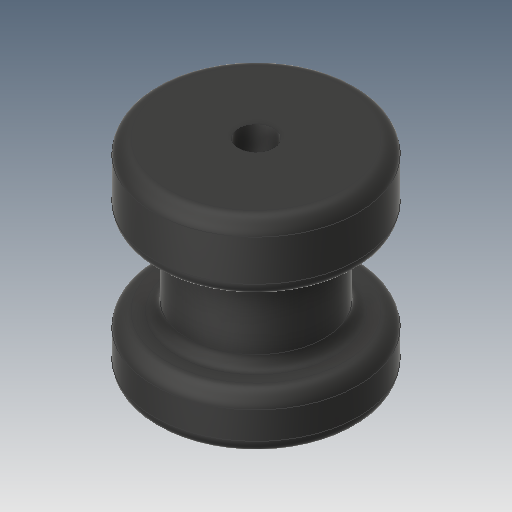
# Autodesk Inventor part: End_Effector_Coupler
Saved by Autodesk Inventor 2020.3 (Build 243373000, 373)
## iProperties
Created: 2021-08-25
Part Number: End_Effector_Coupler
Material: ABS Plastic
Document SubType Name: Modeling
Designer: justi
Density: 1.06 g/cm^3
Appearance: Smooth - Black
Mass: 16.3412 g
Surface Area: 49.2182 cm^2
Volume: 15.4162 cm^3
Author: justi
Autodesk Inventor part; units mm, degrees
ref_plane "YZ Plane" through (0, 0, 0) normal (1, 0, 0) x (0, 1, 0)
ref_plane "XZ Plane" through (0, 0, 0) normal (0, 1, 0) x (-1, 0, 0)
sketch "Sketch2" plane through (0, 0, 0) normal (0, 0, 1) x (1, 0, 0)
  line L0 (0, -14.5) -> (0, 15.5)
  line L1 (0, 15.5) -> (-15, 15.5)
  line L2 (0, -14.5) -> (-15, -14.5)
  line L3 (-15, 15.5) -> (-15, 5.5)
  line L4 (-15, 5.5) -> (-10, 5.5)
  line L5 (-10, 5.5) -> (-10, -6.5)
  line L6 (-10, -6.5) -> (-15, -6.5)
  line L7 (-15, -6.5) -> (-15, -14.5)
  line L8 (-10, -0.5) -> (-2.7173, -0.5)
  point P0 (0, 0)
  dimension "d9" = 30
  dimension "d10" = 15
  dimension "d11" = 15
  dimension "d12" = 10
  dimension "d13" = 5
  dimension "d14" = 12
  constraints: 18 end point, 4 horizontal, 3 perpendicular, 2 vertical, 1 midpoint
  measures "d9" distance of L0.start L0.end
  measures "d10" distance of L0.end L1.end
  measures "d11" distance of L0.start L2.end
  measures "d12" distance of L1.end L3.end
  measures "d13" distance of L3.end L4.end
  measures "d14" distance of L4.end L5.end
revolve "Revolution1" add sketch "Sketch2" angle 360 about axis through (0, -14.5, 0) along (0, 1, 0)
sketch "Sketch3" plane through (0, 15.5, 0) normal (0, 1, 0) x (1, 0, 0)
  circle A0 centre (0, 0) radius 2.6
  dimension "d16" = 5.2
  constraints: 1 centre point, 1 coincident
  measures "d16" diameter of A0
extrude "Extrusion1" cut sketch "Sketch3" against normal blind 17
ref_plane "Work Plane1" through (0, 0, -15) normal (0, 0, 1) x (1, 0, 0)
sketch "Sketch4" plane through (0, 0, -15) normal (0, 0, 1) x (1, 0, 0)
  line L0 (15, 15.5) -> (-15, 15.5) projected
  line L1 (0, 15.5) -> (0, 0) construction
  line L2 (-2.6, 15.5) -> (-2.6, -1.5) projected
  circle A0 centre (0, 7.75) radius 1.6
  circle A1 centre (0, 7.75) radius 1.6
  dimension "d20" = 3.2
  dimension "d33" = 3.2
  constraints: 2 centre point, 2 end point, 2 midpoint, 1 coincident, 1 parallel
  measures "d20" diameter of A0
  measures "d33" diameter of A1
extrude "Extrusion2" cut sketch "Sketch4" along normal up to surface round surface about axis through (0, 15.5, 0) along (0, -1, 0) radius 2.6 far side no
sketch "Sketch5" plane through (0, -14.5, 0) normal (0, -1, 0) x (1, 0, 0)
  line L0 (5, 5) -> (-5, 5) construction
  line L1 (-5, 5) -> (-5, -5) construction
  line L2 (-5, -5) -> (5, -5) construction
  line L3 (5, -5) -> (5, 5) construction
  line L4 (5, 5) -> (-5, -5) construction
  line L5 (-5, 5) -> (5, -5) construction
  circle A0 centre (5, -5) radius 2.4
  circle A1 centre (-5, 5) radius 2.4
  point P0 (0, 0)
  dimension "d23" = 10
  dimension "d24" = 10
  dimension "d26" = 4.8
  dimension "d27" = 4.8
  constraints: 12 end point, 2 centre point, 2 coincident, 2 midpoint, 2 parallel, 1 horizontal, 1 perpendicular
  measures "d23" distance of L2.end L1.end
  measures "d24" distance of L1.end L0.end
  measures "d26" diameter of A0
  measures "d27" diameter of A1
extrude "Extrusion3" cut sketch "Sketch5" against normal blind 10
fillet "Fillet1" radius 2 4 edges at (15, 5.5, 0) (15, -6.5, 0) (15, 15.5, 0) (15, -14.5, 0)
sketch "Sketch7" plane through (0, 0, -15) normal (0, 0, 1) x (1, 0, 0)
  point P0 (0, 0)
extrude "Extrusion4" cut sketch "Sketch4" along normal up to surface round surface about axis through (0, 15.5, 0) along (0, -1, 0) radius 2.6 far side no
fillet "Fillet2" radius 1.5 2 edges at (10, -6.5, 0) (10, 5.5, 0)
fillet "Fillet3" radius 0.5 2 edges at (-7.4, -14.5, 5) (2.6, -14.5, -5)
equation "\"d11\" = d10"
body "Solid1"
